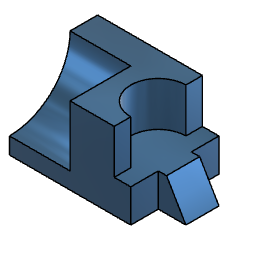
3d 1 v1 (Autodesk Fusion 360 design; units mm, degrees)
Autodesk Fusion 360 part; units mm, degrees
note: some values were not read from the file. Set by a fixed rule: which sketch regions a step uses.
sketch "Sketch1" plane through (0, 0, 0) normal (0, 0, 1) x (1, 0, 0)
  line L0 (0, 0) -> (88, 0)
  line L1 (88, 0) -> (88, 24)
  line L2 (88, 24) -> (76, 24)
  line L3 (76, 24) -> (76, 56)
  line L4 (76, 56) -> (0, 56)
  line L5 (0, 56) -> (0, 0)
  dimension "d1" = 88
  dimension "d2" = 24
  dimension "d3" = 12
  dimension "d4" = 32
  constraint coincident L0.start L5.end
  constraint horizontal L0
  constraint perpendicular L0 L1
  constraint perpendicular L1 L2
  constraint perpendicular L2 L3
  constraint perpendicular L3 L4
  constraint perpendicular L4 L5
  measures "d1" distance of L0.start L0.end
  measures "d2" distance of L0.end L1.end
  measures "d3" distance of L1.end L2.end
  measures "d4" distance of L2.end L3.end
extrude "Extrude1" add sketch "Sketch1" along normal mid plane 64
sketch "Sketch2" plane through (0, 0, 0) normal (0, 0, 1) x (1, 0, 0)
  line L0 (88, 0) -> (108, 0)
  line L1 (108, 0) -> (94, 24)
  line L2 (94, 24) -> (88, 24)
  line L3 (88, 24) -> (88, 0)
  point P0 (88, 24)
  point P1 (88, 0)
  dimension "d7" = 20
  dimension "d8" = 6
  constraint horizontal L0
  constraint parallel L0 L2
  constraint perpendicular L0 L3
  constraint coincident P0 L2.end
  constraint coincident L0.start L3.end
  measures "d7" distance of L0.start L0.end
  measures "d8" distance of L1.end P0
extrude "Extrude2" add sketch "Sketch2" along normal mid plane 24
sketch "Sketch3" plane through (0, 56, 0) normal (0, 1, 0) x (-1, 0, 0)
  line L0 (0, -32) -> (0, 32)
  line L1 (0, 32) -> (-76, 32)
  line L2 (-76, 32) -> (-76, -32)
  line L3 (-76, -32) -> (0, -32)
  circle A0 centre (-76, 0) radius 20
  dimension "d11" = 40
  constraint midpoint L2 A0.centre
  measures "d11" diameter of A0
extrude "Extrude3" cut sketch "Sketch3" against normal blind 32 contours L2 A0 picked at (-67.9161, 5.5729)
sketch "Sketch4" plane through (0, 0, 0) normal (-1, 0, 0) x (0, 0, 1)
  line L0 (-32, 0) -> (32, 0)
  line L1 (32, 0) -> (32, 56)
  line L2 (32, 56) -> (-32, 56)
  line L3 (-32, 56) -> (-32, 0)
  circle A0 centre (32, 56) radius 44
  dimension "d14" = 88
  constraint coincident L1.end L2.start
  measures "d14" diameter of A0
extrude "Extrude4" cut sketch "Sketch4" against normal blind 44 contours L1 L2 A0 picked at (29.9127, 26.816)
